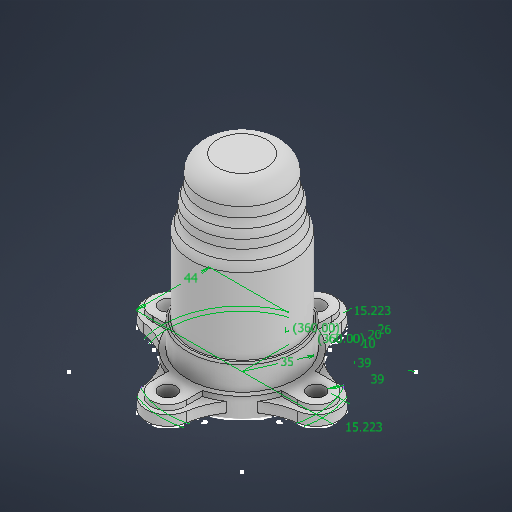
# Autodesk Inventor part: Day02_Task03
Saved by Autodesk Inventor 2026.3 (Build 303398000, 398)
## iProperties
Created: 2026-08-05
Part Number: Day02_Task03
Material: 일반
Document SubType Name: Modeling
Designer: hojin
Density: 1 g/cm^3
Appearance: 기본값
Author: hojin
Autodesk Inventor part; units mm, degrees
ref_plane "YZ Plane" through (0, 0, 0) normal (1, 0, 0) x (0, 1, 0)
ref_plane "XZ Plane" through (0, 0, 0) normal (0, 1, 0) x (-1, 0, 0)
ref_plane "XY Plane" through (0, 0, 0) normal (0, 0, 1) x (1, 0, 0)
sketch "스케치1" plane through (0, 0, 0) normal (0, 0, 1) x (1, 0, 0)
  line L0 (0, 0) -> (32, 0)
  line L1 (0, 112) -> (0, 0)
  line L2 (0, 15) -> (21, 15)
  line L3 (0, 69) -> (24, 69)
  line L4 (0, 84) -> (21, 84)
  line L5 (0, 89) -> (17.5, 89)
  line L6 (0, 101) -> (16, 101)
  line L7 (0, 104) -> (10.5, 104)
  line L8 (0, 112) -> (14.5, 112)
  line L9 (10.5, 104) -> (10.5, 101)
  line L10 (16, 101) -> (16, 89)
  line L11 (17.5, 89) -> (17.5, 84)
  line L12 (21, 84) -> (21, 69)
  line L13 (24, 69) -> (24, 15)
  line L14 (24, 15) -> (21, 15)
  line L15 (21, 15) -> (21, 0)
  line L16 (30, 72) -> (30, 27)
  line L17 (32, 0) -> (32, 26)
  line L18 (31, 27) -> (30, 27)
  arc A0 (24.5, 102) -> (14.5, 112) centre (14.5, 102) ccw
  arc A1 (32, 26) -> (31, 27) centre (31, 26) ccw
  arc A2 (27, 87) -> (25.75, 91.5758) centre (18, 87) ccw
  arc A3 (24.5, 96.1515) -> (25.75, 91.5758) centre (33.5, 96.1515) ccw
  line L19 (24.5, 102) -> (24.5, 96.1515)
  line L20 (27, 87) -> (27, 81.9499)
  arc A4 (27, 81.9499) -> (28.5, 76.9749) centre (36, 81.9499) ccw
  arc A5 (30, 72) -> (28.5, 76.9749) centre (21, 72) ccw
  point P0 (32, 27)
  dimension "d0" = 32
  dimension "d10" = 112
  dimension "d11" = 21
  dimension "d13" = 15
  dimension "d14" = 24
  dimension "d15" = 54
  dimension "d16" = 21
  dimension "d17" = 15
  dimension "d18" = 17.5
  dimension "d19" = 5
  dimension "d20" = 16
  dimension "d21" = 12
  dimension "d22" = 10.5
  dimension "d23" = 3
  dimension "d28" = 30
  dimension "d29" = 27
  dimension "d30" = 10
  dimension "d31" = 1
  dimension "d36" = 9
  dimension "d37" = 9
  dimension "d38" = 27
  dimension "d42" = 24.5
  dimension "d43" = 25
  dimension "d44" = 9
  dimension "d45" = 9
  dimension "d46" = 40
  constraints: 42 end point, 12 point on circle, 10 tangent, 8 horizontal, 8 perpendicular, 7 point on line, 6 centre point, 6 vertical alignment, 5 vertical
  measures "d0" distance of L0.end L0.start
  measures "d10" distance of L0.start L1.start
  measures "d11" distance of L2.start L2.end
  measures "d13" distance of L0.start L2.start
  measures "d14" distance of L3.start L3.end
  measures "d15" distance of L2.start L3.start
  measures "d16" distance of L4.start L4.end
  measures "d17" distance of L3.start L4.start
  measures "d18" distance of L5.start L5.end
  measures "d19" distance of L5.start L4.start
  measures "d20" distance of L6.start L6.end
  measures "d21" distance of L5.start L6.start
  measures "d22" distance of L7.start L7.end
  measures "d23" vertical distance of L6.end L7.end
  measures "d28" horizontal distance of L1.start L16.start
  measures "d29" distance of L0.end point (32, 27)
  measures "d30" radius of A0
  measures "d31" radius of A1
  measures "d36" radius of A2
  measures "d37" radius of A3
  measures "d38" horizontal distance of L1.start L20.start
  measures "d42" horizontal distance of L1.start L19.end
  measures "d43" vertical distance of L1.start L20.start
  measures "d44" radius of A5
  measures "d45" radius of A4
  measures "d46" vertical distance of L1.start L16.start
revolve "회전1" add sketch "스케치1" angle 360 about axis through (0, 112, 0) along (0, -1, 0) contours L15 L14 L13 L3 L12 L4 L11 L5 L10 L6 L9 L7 L1 L8 A0 L19 A3 A2 L20 A4 A5 L16 L18 A1 L17 L0
sketch "스케치2" plane through (0, 0, 0) normal (0, 1, 0) x (-1, 0, 0)
  circle A0 centre (0, -44) radius 5
  arc A1 (-9.9352, -42.8636) -> (9.9352, -42.8636) centre (0, -44) ccw
  arc A2 (-10, -35.6934) -> (10, -35.6934) centre (0, -44) ccw
  line L0 (-10, -44) -> (-10, -33.541)
  line L1 (10, -44) -> (10, -33.541)
  circle A3 centre (44, 0) radius 5
  arc A4 (42.8636, -9.9352) -> (42.8636, 9.9352) centre (44, 0) ccw
  arc A5 (35.6934, -10) -> (35.6934, 10) centre (44, 0) ccw
  line L2 (44, -10) -> (33.541, -10)
  line L3 (44, 10) -> (33.541, 10)
  circle A6 centre (0, 44) radius 5
  arc A7 (9.9352, 42.8636) -> (-9.9352, 42.8636) centre (0, 44) ccw
  arc A8 (10, 35.6934) -> (-10, 35.6934) centre (0, 44) ccw
  line L4 (10, 44) -> (10, 33.541)
  line L5 (-10, 44) -> (-10, 33.541)
  circle A9 centre (-44, 0) radius 5
  arc A10 (-42.8636, 9.9352) -> (-42.8636, -9.9352) centre (-44, 0) ccw
  arc A11 (-35.6934, 10) -> (-35.6934, -10) centre (-44, 0) ccw
  line L6 (-44, 10) -> (-33.541, 10)
  line L7 (-44, -10) -> (-33.541, -10)
  arc A12 (-33.541, -10) -> (-10, -33.541) centre (0, 0) ccw
  arc A13 (-10, 33.541) -> (-33.541, 10) centre (0, 0) ccw
  arc A14 (10, -33.541) -> (33.541, -10) centre (0, 0) ccw
  arc A15 (33.541, 10) -> (10, 33.541) centre (0, 0) ccw
  arc A16 (-12.8655, -45.8655) -> (-19.5652, -29.0208) centre (-51.4618, -51.4618) ccw
  arc A17 (-29.0208, -19.5652) -> (-45.8655, -12.8655) centre (-51.4618, -51.4618) ccw
  arc A18 (-42.8636, -9.9352) -> (-42.8486, -10) centre (0, 0) ccw
  arc A19 (-42.8486, 10) -> (-42.8636, 9.9352) centre (0, 0) ccw
  arc A20 (-9.9352, 42.8636) -> (-10, 42.8486) centre (0, 0) ccw
  arc A21 (-13.672, 41.822) -> (-41.822, 13.672) centre (0, 0) ccw
  arc A22 (10, 42.8486) -> (9.9352, 42.8636) centre (0, 0) ccw
  arc A23 (42.8636, 9.9352) -> (42.8486, 10) centre (0, 0) ccw
  arc A24 (41.822, 13.672) -> (13.672, 41.822) centre (0, 0) ccw
  arc A25 (42.8486, -10) -> (42.8636, -9.9352) centre (0, 0) ccw
  arc A26 (9.9352, -42.8636) -> (10, -42.8486) centre (0, 0) ccw
  arc A27 (13.672, -41.822) -> (41.822, -13.672) centre (0, 0) ccw
  arc A28 (-41.822, -13.672) -> (-13.672, -41.822) centre (0, 0) ccw
  arc A29 (-10, -42.8486) -> (-9.9352, -42.8636) centre (0, 0) ccw
  arc A30 (45.8655, -12.8655) -> (29.0208, -19.5652) centre (51.4618, -51.4618) ccw
  arc A31 (19.5652, -29.0208) -> (12.8655, -45.8655) centre (51.4618, -51.4618) ccw
  arc A32 (12.8655, 45.8655) -> (19.5652, 29.0208) centre (51.4618, 51.4618) ccw
  arc A33 (29.0208, 19.5652) -> (45.8655, 12.8655) centre (51.4618, 51.4618) ccw
  arc A34 (-45.8655, 12.8655) -> (-29.0208, 19.5652) centre (-51.4618, 51.4618) ccw
  arc A35 (-19.5652, 29.0208) -> (-12.8655, 45.8655) centre (-51.4618, 51.4618) ccw
  point P0 (-37.0484, -15.223)
  point P1 (-15.223, -37.0484)
  point P2 (37.0484, -15.223)
  point P3 (15.223, -37.0484)
  point P4 (15.223, 37.0484)
  point P5 (37.0484, 15.223)
  point P6 (-37.0484, 15.223)
  point P7 (-15.223, 37.0484)
  point P8 (-29.0208, 19.5652)
  point P9 (-45.8655, 12.8655)
  point P10 (12.8655, -45.8655)
  point P11 (19.5652, -29.0208)
  point P12 (45.8655, 12.8655)
  point P13 (29.0208, 19.5652)
  point P14 (29.0208, -19.5652)
  point P15 (45.8655, -12.8655)
  point P16 (-12.8655, 45.8655)
  point P17 (-19.5652, 29.0208)
  point P18 (19.5652, 29.0208)
  point P19 (12.8655, 45.8655)
  dimension "d51" = 10
  dimension "d52" = 20
  dimension "d53" = 26
  dimension "d58" = 360
  dimension "d60" = 35
  dimension "d61" = 44
  dimension "d65" = 39
  dimension "d66" = 39
  dimension "d67" = 15.223
  dimension "d68" = 15.223
  dimension "d71" = 360
  constraints: 86 point on circle, 36 centre point, 16 end point, 16 point on line, 10 coincident, 2 tangent, 2 vertical, 1 vertical alignment, 106 other
  measures "d51" diameter of A0
  measures "d52" diameter of A1
  measures "d53" diameter of A2
  measures "d60" radius of A12
  measures "d61" distance of A0.centre point (0, 0)
  measures "d65" radius of A16
  measures "d66" radius of A17
  measures "d67" vertical distance of point (-37.048, -15.223) point (0, 0)
  measures "d68" horizontal distance of point (0, 0) point (-15.223, -37.048)
extrude "돌출1" cut sketch "스케치2" along normal blind 12 contours A29 L0 A12 L7 A18 A10 A19 L6 A13 L5 A20 A7 A22 L4 A15 L3 A23 A4 A25 L2 A14 L1 A26 A1
extrude "돌출2" add sketch "스케치2" along normal blind 12 contours A29 L0 A12 L7 A18 A10 A19 L6 A13 L5 A20 A7 A22 L4 A15 L3 A23 A4 A25 L2 A14 L1 A26 A1
extrude "돌출3" add sketch "스케치2" along normal blind 9 contours A1 L1 A2 L0 | A2 A16 A12 L0 | L1 A14 A31 A2 | A17 A11 L7 A12 | A30 A14 L2 A5 | A11 L6 A10 L7 | A5 L2 A4 L3 | A34 A13 L6 A11 | A5 L3 A15 A33 | A35 A8 L5 A13 | A32 A15 L4 A8 | A8 L4 A7 L5
extrude "돌출4" cut sketch "스케치2" along normal blind 3 contours A1 L1 A2 L0 | A2 A16 A12 L0 | L1 A14 A31 A2 | A17 A11 L7 A12 | A30 A14 L2 A5 | A11 L6 A10 L7 | A5 L2 A4 L3 | A34 A13 L6 A11 | A5 L3 A15 A33 | A35 A8 L5 A13 | A32 A15 L4 A8 | A8 L4 A7 L5
